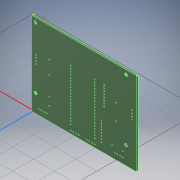
# Autodesk Inventor part: low_level_contoller_board2.brdКонтур
Saved by Autodesk Inventor 2022 (Build 260153000, 153)
## iProperties
Created: 2023-01-22
Part Number: low_level_contoller_board2.brdКонтур
Material: Типовые
Document SubType Name: Modeling
Designer: Иван Петров
Density: 1 g/cm^3
Appearance: Контур панели
Author: Иван Петров
Autodesk Inventor part; units mm, degrees
ref_plane "YZ Plane" through (0, 0, 0) normal (1, 0, 0) x (0, 1, 0)
ref_plane "XZ Plane" through (0, 0, 0) normal (0, 1, 0) x (-1, 0, 0)
ref_plane "XY Plane" through (0, 0, 0) normal (0, 0, 1) x (1, 0, 0)
sketch "Эскиз1" plane through (0, 0, 0) normal (0, 0, 1) x (1, 0, 0)
  line L0 (-0.6, -0.6) -> (-0.6, -78.4)
  line L1 (-0.6, -78.4) -> (-0.5796, -78.5553)
  line L2 (-0.5796, -78.5553) -> (-0.5196, -78.7)
  line L3 (-0.5196, -78.7) -> (-0.4243, -78.8243)
  line L4 (-0.4243, -78.8243) -> (-0.3, -78.9196)
  line L5 (-0.3, -78.9196) -> (-0.1553, -78.9796)
  line L6 (-0.1553, -78.9796) -> (0, -79)
  line L7 (0, -79) -> (98.8, -79)
  line L8 (98.8, -79) -> (98.9553, -78.9796)
  line L9 (98.9553, -78.9796) -> (99.1, -78.9196)
  line L10 (99.1, -78.9196) -> (99.2243, -78.8243)
  line L11 (99.2243, -78.8243) -> (99.3196, -78.7)
  line L12 (99.3196, -78.7) -> (99.3796, -78.5553)
  line L13 (99.3796, -78.5553) -> (99.4, -78.4)
  line L14 (99.4, -78.4) -> (99.4, -0.6)
  line L15 (99.4, -0.6) -> (99.3796, -0.4447)
  line L16 (99.3796, -0.4447) -> (99.3196, -0.3)
  line L17 (99.3196, -0.3) -> (99.2243, -0.1757)
  line L18 (99.2243, -0.1757) -> (99.1, -0.0804)
  line L19 (99.1, -0.0804) -> (98.9553, -0.0204)
  line L20 (98.9553, -0.0204) -> (98.8, 0)
  line L21 (98.8, 0) -> (0, 0)
  line L22 (0, 0) -> (-0.1553, -0.0204)
  line L23 (-0.1553, -0.0204) -> (-0.3, -0.0804)
  line L24 (-0.3, -0.0804) -> (-0.4243, -0.1757)
  line L25 (-0.4243, -0.1757) -> (-0.5196, -0.3)
  line L26 (-0.5196, -0.3) -> (-0.5796, -0.4447)
  line L27 (-0.5796, -0.4447) -> (-0.6, -0.6)
  line L28 (90.775, -62) -> (90.7632, -61.8205)
  line L29 (90.7632, -61.8205) -> (90.7281, -61.6441)
  line L30 (90.7281, -61.6441) -> (90.5908, -61.3125)
  line L31 (90.5908, -61.3125) -> (90.3723, -61.0277)
  line L32 (90.3723, -61.0277) -> (90.0875, -60.8092)
  line L33 (90.0875, -60.8092) -> (89.7559, -60.6719)
  line L34 (89.7559, -60.6719) -> (89.4, -60.625)
  line L35 (89.4, -60.625) -> (89.0441, -60.6719)
  line L36 (89.0441, -60.6719) -> (88.7125, -60.8092)
  line L37 (88.7125, -60.8092) -> (88.4277, -61.0277)
  line L38 (88.4277, -61.0277) -> (88.2092, -61.3125)
  line L39 (88.2092, -61.3125) -> (88.0719, -61.6441)
  line L40 (88.0719, -61.6441) -> (88.025, -62)
  line L41 (88.025, -62) -> (88.0719, -62.3559)
  line L42 (88.0719, -62.3559) -> (88.2092, -62.6875)
  line L43 (88.2092, -62.6875) -> (88.4277, -62.9723)
  line L44 (88.4277, -62.9723) -> (88.7125, -63.1908)
  line L45 (88.7125, -63.1908) -> (89.0441, -63.3281)
  line L46 (89.0441, -63.3281) -> (89.4, -63.375)
  line L47 (89.4, -63.375) -> (89.7559, -63.3281)
  line L48 (89.7559, -63.3281) -> (90.0875, -63.1908)
  line L49 (90.0875, -63.1908) -> (90.3723, -62.9723)
  line L50 (90.3723, -62.9723) -> (90.5908, -62.6875)
  line L51 (90.5908, -62.6875) -> (90.7281, -62.3559)
  line L52 (90.7281, -62.3559) -> (90.775, -62)
  line L53 (4.775, -62) -> (4.7632, -61.8205)
  line L54 (4.7632, -61.8205) -> (4.7281, -61.6441)
  line L55 (4.7281, -61.6441) -> (4.5908, -61.3125)
  line L56 (4.5908, -61.3125) -> (4.3723, -61.0277)
  line L57 (4.3723, -61.0277) -> (4.0875, -60.8092)
  line L58 (4.0875, -60.8092) -> (3.7559, -60.6719)
  line L59 (3.7559, -60.6719) -> (3.4, -60.625)
  line L60 (3.4, -60.625) -> (3.0441, -60.6719)
  line L61 (3.0441, -60.6719) -> (2.7125, -60.8092)
  line L62 (2.7125, -60.8092) -> (2.4277, -61.0277)
  line L63 (2.4277, -61.0277) -> (2.2092, -61.3125)
  line L64 (2.2092, -61.3125) -> (2.0719, -61.6441)
  line L65 (2.0719, -61.6441) -> (2.025, -62)
  line L66 (2.025, -62) -> (2.0719, -62.3559)
  line L67 (2.0719, -62.3559) -> (2.2092, -62.6875)
  line L68 (2.2092, -62.6875) -> (2.4277, -62.9723)
  line L69 (2.4277, -62.9723) -> (2.7125, -63.1908)
  line L70 (2.7125, -63.1908) -> (3.0441, -63.3281)
  line L71 (3.0441, -63.3281) -> (3.4, -63.375)
  line L72 (3.4, -63.375) -> (3.7559, -63.3281)
  line L73 (3.7559, -63.3281) -> (4.0875, -63.1908)
  line L74 (4.0875, -63.1908) -> (4.3723, -62.9723)
  line L75 (4.3723, -62.9723) -> (4.5908, -62.6875)
  line L76 (4.5908, -62.6875) -> (4.7281, -62.3559)
  line L77 (4.7281, -62.3559) -> (4.775, -62)
  line L78 (4.775, -4) -> (4.7632, -3.8205)
  line L79 (4.7632, -3.8205) -> (4.7281, -3.6441)
  line L80 (4.7281, -3.6441) -> (4.5908, -3.3125)
  line L81 (4.5908, -3.3125) -> (4.3723, -3.0277)
  line L82 (4.3723, -3.0277) -> (4.0875, -2.8092)
  line L83 (4.0875, -2.8092) -> (3.7559, -2.6719)
  line L84 (3.7559, -2.6719) -> (3.4, -2.625)
  line L85 (3.4, -2.625) -> (3.0441, -2.6719)
  line L86 (3.0441, -2.6719) -> (2.7125, -2.8092)
  line L87 (2.7125, -2.8092) -> (2.4277, -3.0277)
  line L88 (2.4277, -3.0277) -> (2.2092, -3.3125)
  line L89 (2.2092, -3.3125) -> (2.0719, -3.6441)
  line L90 (2.0719, -3.6441) -> (2.025, -4)
  line L91 (2.025, -4) -> (2.0719, -4.3559)
  line L92 (2.0719, -4.3559) -> (2.2092, -4.6875)
  line L93 (2.2092, -4.6875) -> (2.4277, -4.9723)
  line L94 (2.4277, -4.9723) -> (2.7125, -5.1908)
  line L95 (2.7125, -5.1908) -> (3.0441, -5.3281)
  line L96 (3.0441, -5.3281) -> (3.4, -5.375)
  line L97 (3.4, -5.375) -> (3.7559, -5.3281)
  line L98 (3.7559, -5.3281) -> (4.0875, -5.1908)
  line L99 (4.0875, -5.1908) -> (4.3723, -4.9723)
  line L100 (4.3723, -4.9723) -> (4.5908, -4.6875)
  line L101 (4.5908, -4.6875) -> (4.7281, -4.3559)
  line L102 (4.7281, -4.3559) -> (4.775, -4)
  line L103 (90.775, -4) -> (90.7632, -3.8205)
  line L104 (90.7632, -3.8205) -> (90.7281, -3.6441)
  line L105 (90.7281, -3.6441) -> (90.5908, -3.3125)
  line L106 (90.5908, -3.3125) -> (90.3723, -3.0277)
  line L107 (90.3723, -3.0277) -> (90.0875, -2.8092)
  line L108 (90.0875, -2.8092) -> (89.7559, -2.6719)
  line L109 (89.7559, -2.6719) -> (89.4, -2.625)
  line L110 (89.4, -2.625) -> (89.0441, -2.6719)
  line L111 (89.0441, -2.6719) -> (88.7125, -2.8092)
  line L112 (88.7125, -2.8092) -> (88.4277, -3.0277)
  line L113 (88.4277, -3.0277) -> (88.2092, -3.3125)
  line L114 (88.2092, -3.3125) -> (88.0719, -3.6441)
  line L115 (88.0719, -3.6441) -> (88.025, -4)
  line L116 (88.025, -4) -> (88.0719, -4.3559)
  line L117 (88.0719, -4.3559) -> (88.2092, -4.6875)
  line L118 (88.2092, -4.6875) -> (88.4277, -4.9723)
  line L119 (88.4277, -4.9723) -> (88.7125, -5.1908)
  line L120 (88.7125, -5.1908) -> (89.0441, -5.3281)
  line L121 (89.0441, -5.3281) -> (89.4, -5.375)
  line L122 (89.4, -5.375) -> (89.7559, -5.3281)
  line L123 (89.7559, -5.3281) -> (90.0875, -5.1908)
  line L124 (90.0875, -5.1908) -> (90.3723, -4.9723)
  line L125 (90.3723, -4.9723) -> (90.5908, -4.6875)
  line L126 (90.5908, -4.6875) -> (90.7281, -4.3559)
  line L127 (90.7281, -4.3559) -> (90.775, -4)
  circle A0 centre (52.07, -76.2) radius 0.51
  circle A1 centre (54.61, -76.2) radius 0.51
  circle A2 centre (57.15, -76.2) radius 0.51
  circle A3 centre (59.69, -76.2) radius 0.51
  circle A4 centre (36.83, -76.2) radius 0.51
  circle A5 centre (39.37, -76.2) radius 0.51
  circle A6 centre (41.91, -76.2) radius 0.51
  circle A7 centre (44.45, -76.2) radius 0.51
  circle A8 centre (95.12, -30.48) radius 0.51
  circle A9 centre (95.12, -33.02) radius 0.51
  circle A10 centre (95.12, -35.56) radius 0.51
  circle A11 centre (95.12, -38.1) radius 0.51
  circle A12 centre (3.81, -38.1) radius 0.51
  circle A13 centre (3.81, -35.56) radius 0.51
  circle A14 centre (3.81, -33.02) radius 0.51
  circle A15 centre (3.81, -30.48) radius 0.51
  circle A16 centre (86.36, -73.66) radius 0.51
  circle A17 centre (83.82, -73.66) radius 0.51
  circle A18 centre (81.28, -73.66) radius 0.51
  circle A19 centre (78.74, -73.66) radius 0.51
  circle A20 centre (13.97, -73.66) radius 0.51
  circle A21 centre (11.43, -73.66) radius 0.51
  circle A22 centre (8.89, -73.66) radius 0.51
  circle A23 centre (6.35, -73.66) radius 0.51
  circle A24 centre (66.04, -63.5) radius 0.51
  circle A25 centre (66.04, -66.04) radius 0.51
  circle A26 centre (66.04, -68.58) radius 0.51
  circle A27 centre (66.04, -71.12) radius 0.51
  circle A28 centre (66.04, -53.34) radius 0.51
  circle A29 centre (66.04, -55.88) radius 0.51
  circle A30 centre (66.04, -58.42) radius 0.51
  circle A31 centre (66.04, -60.96) radius 0.51
  circle A32 centre (68.58, -22.86) radius 0.6
  circle A33 centre (68.58, -25.4) radius 0.6
  circle A34 centre (68.58, -27.94) radius 0.6
  circle A35 centre (68.58, -30.48) radius 0.6
  circle A36 centre (68.58, -33.02) radius 0.6
  circle A37 centre (68.58, -35.56) radius 0.6
  circle A38 centre (68.58, -38.1) radius 0.6
  circle A39 centre (68.58, -40.64) radius 0.6
  circle A40 centre (36.83, -33.02) radius 0.5
  circle A41 centre (36.83, -35.56) radius 0.5
  circle A42 centre (36.83, -38.1) radius 0.5
  circle A43 centre (36.83, -40.64) radius 0.5
  circle A44 centre (36.83, -27.94) radius 0.5
  circle A45 centre (36.83, -43.18) radius 0.5
  circle A46 centre (36.83, -45.72) radius 0.5
  circle A47 centre (36.83, -25.4) radius 0.5
  circle A48 centre (59.69, -68.58) radius 0.5
  circle A49 centre (36.83, -48.26) radius 0.5
  circle A50 centre (36.83, -50.8) radius 0.5
  circle A51 centre (36.83, -53.34) radius 0.5
  circle A52 centre (36.83, -55.88) radius 0.5
  circle A53 centre (36.83, -58.42) radius 0.5
  circle A54 centre (36.83, -60.96) radius 0.5
  circle A55 centre (36.83, -63.5) radius 0.5
  circle A56 centre (36.83, -66.04) radius 0.5
  circle A57 centre (36.83, -68.58) radius 0.5
  circle A58 centre (36.83, -71.12) radius 0.5
  circle A59 centre (59.69, -43.18) radius 0.5
  circle A60 centre (59.69, -45.72) radius 0.5
  circle A61 centre (59.69, -48.26) radius 0.5
  circle A62 centre (59.69, -50.8) radius 0.5
  circle A63 centre (59.69, -53.34) radius 0.5
  circle A64 centre (59.69, -55.88) radius 0.5
  circle A65 centre (59.69, -58.42) radius 0.5
  circle A66 centre (59.69, -60.96) radius 0.5
  circle A67 centre (59.69, -63.5) radius 0.5
  circle A68 centre (59.69, -66.04) radius 0.5
  circle A69 centre (59.69, -71.12) radius 0.5
  circle A70 centre (59.69, -35.56) radius 0.5
  circle A71 centre (36.83, -30.48) radius 0.5
  circle A72 centre (59.69, -27.94) radius 0.5
  circle A73 centre (59.69, -30.48) radius 0.5
  circle A74 centre (59.69, -40.64) radius 0.5
  circle A75 centre (36.83, -22.86) radius 0.5
  circle A76 centre (59.69, -33.02) radius 0.5
  circle A77 centre (59.69, -22.86) radius 0.5
  circle A78 centre (59.69, -25.4) radius 0.5
  circle A79 centre (59.69, -38.1) radius 0.5
  circle A80 centre (80.01, -46.99) radius 0.5
  circle A81 centre (80.01, -31.75) radius 0.5
  circle A82 centre (16.51, -58.42) radius 0.5
  circle A83 centre (16.51, -66.04) radius 0.5
  circle A84 centre (16.51, -27.94) radius 0.5
  circle A85 centre (16.51, -40.64) radius 0.5
  circle A86 centre (86.36, -68.58) radius 0.5
  circle A87 centre (76.2, -68.58) radius 0.5
  constraints: 256 end point, 88 centre point
extrude "low_level_contoller_board2.brdКонтур" add sketch "Эскиз1" along normal blind 1.6
sketch "Эскиз2" plane through (0, 0, 0) normal (0, 0, -1) x (-1, 0, 0)
  line L0 (-2.2092, -4.6875) -> (-2.0719, -4.3559) projected
  circle A0 centre (-3.4, -4) radius 1.375
  line L1 (-88.025, -62) -> (-88.0719, -61.6441) projected
  circle A1 centre (-89.4, -62) radius 1.375
  point P0 (0, 0)
  constraints: 6 other
